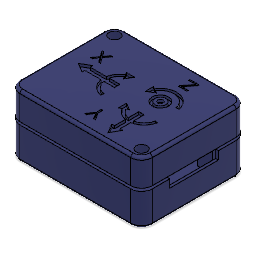
Sensor_Board_Box v9 (Autodesk Fusion 360 design; units mm, degrees)
Autodesk Fusion 360 part; units mm, degrees
sketch "Sketch1" plane through (0, 0, 0) normal (0, 1, 0) x (1, 0, 0)
  line L0 (17.5, -13.25) -> (-17.5, -13.25)
  line L1 (-17.5, -13.25) -> (-17.5, 13.25)
  line L2 (-17.5, 13.25) -> (17.5, 13.25)
  line L3 (17.5, 13.25) -> (17.5, -13.25)
  line L4 (17.5, -13.25) -> (-17.5, 13.25) construction
  line L5 (-17.5, -13.25) -> (17.5, 13.25) construction
  line L6 (-17.5, 13.25) -> (-20.689, 15.6646)
  circle A0 centre (-20.689, 15.6646) radius 1.35
  line L7 (-20.5, 19.5) -> (20.5, 19.5)
  line L8 (24.5, 15.5) -> (24.5, -15.5)
  line L9 (20.5, -19.5) -> (-20.5, -19.5)
  line L10 (-24.5, -15.5) -> (-24.5, 15.5)
  line L11 (-24.5, 19.5) -> (24.5, -19.5) construction
  line L12 (24.5, 19.5) -> (-24.5, -19.5) construction
  line L13 (-24.5, 15.5) -> (-24.5, 12.5)
  line L14 (-24.5, 12.5) -> (-21.5, 12.5)
  line L15 (-20.5, 19.5) -> (-17.5, 19.5)
  line L16 (-17.5, 19.5) -> (-17.5, 16.5)
  arc A1 (-21.5, 12.5) -> (-17.5, 16.5) centre (-21.5, 16.5) ccw
  arc A2 (-20.5, 19.5) -> (-24.5, 15.5) centre (-20.5, 15.5) ccw
  line L17 (24.5, -12.5) -> (21.5, -12.5)
  arc A3 (21.5, -12.5) -> (17.5, -16.5) centre (21.5, -16.5) ccw
  circle A4 centre (20.689, -15.6646) radius 1.35
  line L18 (17.5, -19.5) -> (17.5, -16.5)
  arc A5 (20.5, -19.5) -> (24.5, -15.5) centre (20.5, -15.5) ccw
  line L19 (23.5, -12.5) -> (23.5, 14.5)
  line L20 (23.5, 18.5) -> (-23.5, -18.5) construction
  line L21 (-23.5, 18.5) -> (23.5, -18.5) construction
  line L22 (19.5, 18.5) -> (-17.5, 18.5)
  line L23 (-23.5, 12.5) -> (-23.5, -14.5)
  line L24 (-19.5, -18.5) -> (17.5, -18.5)
  arc A6 (23.5, 14.5) -> (19.5, 18.5) centre (19.5, 14.5) ccw
  arc A7 (24.5, 15.5) -> (20.5, 19.5) centre (20.5, 15.5) ccw
  arc A8 (-23.5, -14.5) -> (-19.5, -18.5) centre (-19.5, -14.5) ccw
  arc A9 (-24.5, -15.5) -> (-20.5, -19.5) centre (-20.5, -15.5) ccw
  dimension "d1" = 35
  dimension "d2" = 26.5
  dimension "d3" = 4
  dimension "d4" = 2.7
  dimension "d5" = 49
  dimension "d6" = 39
  dimension "d7" = 7
  dimension "d8" = 3
  dimension "d9" = 7
  dimension "d10" = 3
  dimension "d11" = 4
  dimension "d13" = 180
  dimension "d14" = 47
  dimension "d15" = 37
  dimension "d16" = 4
  dimension "d17" = 4
  dimension "d18" = 4
  dimension "d19" = 4
  constraint perpendicular L0 L1
  constraint parallel L0 L2
  constraint parallel L1 L3
  constraint horizontal L0
  constraint coincident L4 origin
  constraint coincident L5 origin
  constraint parallel L4 L6
  constraint coincident L6.end A0.centre
  constraint perpendicular L7 L8
  constraint parallel L7 L9
  constraint parallel L8 L10
  constraint horizontal L7
  constraint coincident L11 origin
  constraint coincident L12 origin
  constraint perpendicular L7 L13
  constraint perpendicular L13 L14
  constraint perpendicular L13 L15
  constraint perpendicular L15 L16
  constraint tangent L16 A1
  constraint coincident L11.start L15
  constraint coincident L11.start L13
  constraint tangent L15 A2
  constraint tangent L13 A2
  constraint parallel L22 L24
  constraint horizontal L22
  constraint coincident L20 origin
  constraint coincident L21 origin
  constraint coincident L16 L22.end
  constraint coincident L14 L23.start
  constraint coincident L18 L24.end
  constraint coincident L17 L19.start
  constraint tangent L19 A6
  constraint tangent L22 A6
  constraint coincident L12.start L7
  constraint tangent L8 A7
  constraint tangent L7 A7
  constraint coincident L20.end L24
  constraint coincident L20.end L23
  constraint tangent L24 A8
  constraint tangent L23 A8
  constraint coincident L12.end L9
  constraint coincident L12.end L10
  constraint tangent L9 A9
  constraint tangent L10 A9
  measures "d1" distance of L1.end L2.end
  measures "d2" distance of L0.end L1.end
  measures "d3" distance of L1.end L6.end
  measures "d4" diameter of A0
  measures "d5" distance of L11.end L12.end
  measures "d6" distance of L12.start L11.end
  measures "d7" distance of L11.start L13.end
  measures "d8" distance of L13.end L14.end
  measures "d9" distance of L11.start L15.end
  measures "d10" distance of L15.end L16.end
  measures "d11" radius of A2
  measures "d14" distance of L20.end L21.end
  measures "d15" distance of L21.start L20.end
  measures "d16" radius of A6
  measures "d17" radius of A7
  measures "d18" radius of A8
  measures "d19" radius of A9
sketch "Sketch1 (2)" plane through (0, 0, 0) normal (0, 1, 0) x (1, 0, 0) in component "Bottom"
  line L0 (-24.5, 19.5) -> (24.5, -19.5) construction
  line L1 (-23.5, 18.5) -> (23.5, -18.5) construction
  circle A0 centre (-20.689, 15.6646) radius 1.35
  line L2 (-17.5, 13.25) -> (-20.689, 15.6646) construction
  arc A1 (-21.5, 12.5) -> (-17.5, 16.5) centre (-21.5, 16.5) ccw
  line L3 (-17.5, 13.25) -> (17.5, 13.25)
  line L4 (17.5, -13.25) -> (-17.5, 13.25) construction
  line L5 (-17.5, -13.25) -> (-17.5, 13.25)
  line L6 (19.5, 18.5) -> (-17.5, 18.5)
  line L7 (-20.5, 19.5) -> (20.5, 19.5)
  line L8 (24.5, 19.5) -> (-24.5, -19.5) construction
  line L9 (23.5, 18.5) -> (-23.5, -18.5) construction
  line L10 (23.5, -12.5) -> (23.5, 14.5)
  line L11 (24.5, 15.5) -> (24.5, -15.5)
  line L12 (17.5, 13.25) -> (17.5, -13.25)
  arc A2 (21.5, -12.5) -> (17.5, -16.5) centre (21.5, -16.5) ccw
  line L13 (17.5, -13.25) -> (-17.5, -13.25)
  circle A3 centre (20.689, -15.6646) radius 1.35
  arc A4 (20.5, -19.5) -> (24.5, -15.5) centre (20.5, -15.5) ccw
  line L14 (24.5, -12.5) -> (21.5, -12.5)
  line L15 (20.5, -19.5) -> (-20.5, -19.5)
  line L16 (-19.5, -18.5) -> (17.5, -18.5)
  line L17 (17.5, -19.5) -> (17.5, -16.5)
  line L18 (-17.5, -13.25) -> (17.5, 13.25) construction
  line L19 (-23.5, 12.5) -> (-23.5, -14.5)
  line L20 (-24.5, -15.5) -> (-24.5, 15.5)
  line L21 (-24.5, 12.5) -> (-21.5, 12.5)
  arc A5 (-20.5, 19.5) -> (-24.5, 15.5) centre (-20.5, 15.5) ccw
  line L22 (-17.5, 19.5) -> (-17.5, 16.5)
  arc A6 (-24.5, -15.5) -> (-20.5, -19.5) centre (-20.5, -15.5) ccw
  arc A7 (-23.5, -14.5) -> (-19.5, -18.5) centre (-19.5, -14.5) ccw
  arc A8 (23.5, 14.5) -> (19.5, 18.5) centre (19.5, 14.5) ccw
  arc A9 (24.5, 15.5) -> (20.5, 19.5) centre (20.5, 15.5) ccw
  point P0 (-23.5, 18.5)
  point P1 (-24.5, 19.5)
  point P2 (-21.5, 16.5)
  point P3 (-20.689, 15.6646)
  point P4 (-20.689, 15.6646)
  point P5 (-20.5, 15.5)
  point P6 (-17.5, 13.25)
  point P7 (17.5, -13.25)
  point P8 (20.5, -15.5)
  point P9 (20.689, -15.6646)
  point P10 (24.5, -19.5)
  point P11 (23.5, -18.5)
  point P12 (24.5, -15.5)
  point P13 (24.5, -12.5)
  point P14 (23.5, -12.5)
  point P15 (21.5, -12.5)
  point P16 (21.5, -16.5)
  point P17 (20.5, -19.5)
  point P18 (17.5, -18.5)
  point P19 (17.5, -19.5)
  point P20 (-24.5, -19.5)
  point P21 (-21.5, 12.5)
  point P22 (-23.5, 12.5)
  point P23 (-24.5, 15.5)
  point P24 (-17.5, 19.5)
  point P25 (-20.5, 19.5)
  point P26 (-17.5, 18.5)
  point P27 (-17.5, 16.5)
  point P28 (17.5, 13.25)
  point P29 (-17.5, -13.25)
  point P30 (-23.5, -18.5)
  point P31 (17.5, -16.5)
extrude "Extrude1" add sketch "Sketch1 (2)" along normal blind 2 contours A0 | A1 L7 L20 L21 A5 L22 | A1 L6 L10 A2 L14 L16 L17 L19 L21 L22 A7 A8 | L15 L16 L17 L19 L20 L21 A6 A7 | L6 L7 L10 L11 L14 L22 A8 A9 | L11 A2 A4 L14 L15 L17 | L3 L5 L12 L13 | A3 makes body 1 in component "Bottom"
extrude "Extrude2" add sketch "Sketch1 (2)" along normal blind 3 contours A1 L6 L10 A2 L14 L16 L17 L19 L21 L22 A7 A8 bodies 1 in component "Bottom"
extrude "Extrude3" add 1 faces at (23.1667, 2, 13.5) along direction (0, 1, 0) blind 10 on bodies 1 bodies 1 in component "Bottom"
extrude "Extrude4" cut sketch "Sketch1 (2)" along normal blind 29 from surface at 3 contours A0 | A3 bodies 1 in component "Bottom"
sketch "Sketch1 (3)" plane through (0, 0, 0) normal (0, 0, 1) x (1, 0, 0) in component "Top"
  line L0 (17.5, 3) -> (17.5, 2)
  line L1 (17.5, 2) -> (-17.5, 2)
  line L2 (-17.5, 2) -> (-17.5, 3)
  line L3 (-17.5, 3) -> (-23.5, 3)
  line L4 (-23.5, 3) -> (-23.5, 12)
  line L5 (-23.5, 12) -> (-24.5, 12)
  line L6 (-24.5, 12) -> (-24.5, 0)
  line L7 (-24.5, 0) -> (24.5, 0)
  line L8 (24.5, 0) -> (24.5, 12)
  line L9 (24.5, 12) -> (23.5, 12)
  line L10 (23.5, 12) -> (23.5, 3)
  line L11 (23.5, 3) -> (17.5, 3)
  line L12 (0, 2) -> (0, 22) construction
  dimension "d30" = 20
  constraint vertical L12
  constraint midpoint L1 L12.start
  measures "d30" distance of L12.start L12.end
sketch "Sketch2" plane through (0, 12, 0) normal (0, 1, 0) x (-1, 0, 0) in component "Top"
  line L0 (-17.5, -13.25) -> (-17.5, 13.25) construction
  line L1 (-17.5, 13.25) -> (17.5, 13.25) construction
  line L2 (17.5, -13.25) -> (-17.5, -13.25) construction
  line L3 (-23.5, 12.5) -> (-23.5, -14.5) construction
  arc A0 (-23.5, -14.5) -> (-19.5, -18.5) centre (-19.5, -14.5) ccw construction
  line L4 (-19.5, -18.5) -> (17.5, -18.5) construction
  line L5 (17.5, -18.5) -> (17.5, -16.5) construction
  arc A1 (21.5, -12.5) -> (17.5, -16.5) centre (21.5, -16.5) ccw construction
  line L6 (21.5, -12.5) -> (23.5, -12.5) construction
  line L7 (23.5, -12.5) -> (23.5, 14.5) construction
  arc A2 (23.5, 14.5) -> (19.5, 18.5) centre (19.5, 14.5) ccw construction
  line L8 (19.5, 18.5) -> (-17.5, 18.5) construction
  line L9 (-17.5, 18.5) -> (-17.5, 16.5) construction
  arc A3 (-21.5, 12.5) -> (-17.5, 16.5) centre (-21.5, 16.5) ccw construction
  line L10 (-21.5, 12.5) -> (-23.5, 12.5) construction
  circle A4 centre (20.689, -15.6646) radius 1.35 construction
  circle A5 centre (-20.689, 15.6646) radius 1.35 construction
  arc A6 (21.5, -12.5) -> (17.5, -16.5) centre (21.5, -16.5) ccw construction
  line L11 (17.5, -16.5) -> (17.5, -18.5) construction
  line L12 (17.5, -18.5) -> (-19.5, -18.5) construction
  arc A7 (-19.5, -18.5) -> (-23.5, -14.5) centre (-19.5, -14.5) cw construction
  line L13 (-23.5, -14.5) -> (-23.5, 12.5) construction
  line L14 (-23.5, 12.5) -> (-21.5, 12.5) construction
  arc A8 (-21.5, 12.5) -> (-17.5, 16.5) centre (-21.5, 16.5) ccw construction
  line L15 (-17.5, 16.5) -> (-17.5, 18.5) construction
  line L16 (-17.5, 18.5) -> (19.5, 18.5) construction
  arc A9 (19.5, 18.5) -> (23.5, 14.5) centre (19.5, 14.5) cw construction
  line L17 (23.5, 14.5) -> (23.5, -12.5) construction
  line L18 (23.5, -12.5) -> (21.5, -12.5) construction
  line L19 (17.5, 13.25) -> (17.5, -13.25) construction
  line L20 (17.5, -13.25) -> (-17.5, -13.25) construction
  line L21 (-17.5, -13.25) -> (-17.5, 13.25) construction
  line L22 (-17.5, 13.25) -> (17.5, 13.25) construction
  line L23 (20.5, 19.5) -> (-20.5, 19.5)
  arc A10 (-20.5, 19.5) -> (-24.5, 15.5) centre (-20.5, 15.5) ccw
  line L24 (-24.5, 15.5) -> (-24.5, -15.5)
  arc A11 (-24.5, -15.5) -> (-20.5, -19.5) centre (-20.5, -15.5) ccw
  line L25 (-20.5, -19.5) -> (20.5, -19.5)
  arc A12 (20.5, -19.5) -> (24.5, -15.5) centre (20.5, -15.5) ccw
  line L26 (24.5, -15.5) -> (24.5, 15.5)
  arc A13 (24.5, 15.5) -> (20.5, 19.5) centre (20.5, 15.5) ccw
  circle A14 centre (20.689, -15.6646) radius 2
  line L27 (17.5, -18.5) -> (17, -18.5) construction
  line L28 (17, -18.5) -> (17, -18)
  line L29 (23.5, -12.5) -> (23.5, -12) construction
  line L30 (23.5, -12) -> (23, -12)
  line L31 (17.5, -13.25) -> (17.5, -10.75) construction
  line L32 (17.5, -13.25) -> (15, -13.25) construction
  arc A15 (21, -12) -> (17, -16) centre (21, -16) ccw
  line L33 (15, -13.25) -> (17.5, -10.75)
  line L34 (23.5, -12.5) -> (23, -12.5) construction
  line L35 (23, -12.5) -> (23, -12) construction
  line L36 (23, -12) -> (23.5, -12) construction
  line L37 (23.5, -12) -> (23.5, -12.5) construction
  line L38 (23.5, 14.5) -> (23, 14.5) construction
  line L39 (23, 14.5) -> (23, 14) construction
  line L40 (23, 14) -> (23.5, 14) construction
  line L41 (23.5, 14) -> (23.5, 14.5) construction
  line L42 (19.5, 18.5) -> (19, 18.5) construction
  line L43 (19, 18.5) -> (19, 18) construction
  line L44 (19, 18) -> (19.5, 18)
  line L45 (19.5, 18) -> (19.5, 18.5) construction
  arc A16 (23, 14.5) -> (19.5, 18) centre (19.5, 14.5) ccw
  line L46 (21, -12) -> (23, -12)
  line L47 (23, -12) -> (23, 14.5)
  line L48 (17.5, -18.5) -> (17, -18.5) construction
  line L49 (17, -18.5) -> (17, -18) construction
  line L50 (17, -18) -> (17.5, -18) construction
  line L51 (17.5, -18) -> (17.5, -18.5) construction
  line L52 (17, -16) -> (17, -18)
  line L53 (17.5, -10.75) -> (23, -10.75)
  line L54 (15, -13.25) -> (15, -18)
  line L55 (15, -18) -> (17, -18)
  line L56 (-17.5, 0) -> (17.5, 0)
  line L57 (15, 13.25) -> (17.5, 10.75)
  line L58 (17.5, 13.25) -> (15, 13.25) construction
  line L59 (17.5, 13.25) -> (17.5, 10.75) construction
  line L60 (17.5, 10.75) -> (23, 10.75)
  line L61 (15, 13.25) -> (15, 18)
  line L62 (15, 18) -> (19, 18)
  line L63 (23, 0) -> (21, 0) construction
  line L64 (21, 0) -> (21, -10.75)
  line L65 (21, 0) -> (21, 10.75)
  circle A17 centre (-20.689, 15.6646) radius 2
  line L66 (-17, 16) -> (-17, 18)
  arc A18 (-21, 12) -> (-17, 16) centre (-21, 16) ccw
  line L67 (-21, 12) -> (-23, 12)
  line L68 (-23, 12) -> (-23, -14.5)
  arc A19 (-23, -14.5) -> (-19.5, -18) centre (-19.5, -14.5) ccw
  line L69 (-17, 18) -> (15, 18)
  line L70 (-19.5, -18) -> (15, -18)
  line L71 (-17.5, -13.25) -> (-17.5, -8.25) construction
  line L72 (-17.5, -13.25) -> (-12.5, -13.25) construction
  line L73 (-17.5, -8.25) -> (-12.5, -13.25)
  line L74 (-12.5, -13.25) -> (-12.5, -18)
  line L75 (-17.5, -8.25) -> (-23, -8.25)
  line L76 (-17.5, 8.25) -> (-12.5, 13.25)
  line L77 (-17.5, 13.25) -> (-12.5, 13.25) construction
  line L78 (-17.5, 13.25) -> (-17.5, 8.25) construction
  line L79 (-17.5, 8.25) -> (-23, 8.25)
  line L80 (-12.5, 13.25) -> (-12.5, 18)
  line L81 (-23, 0) -> (-21, 0) construction
  line L82 (-12.5, -18) -> (-12.5, -16) construction
  line L83 (-12.5, -16) -> (15, -16)
  line L84 (15, 18) -> (15, 16) construction
  line L85 (15, 16) -> (-12.5, 16)
  line L86 (-21, 0) -> (-21, -8.25)
  line L87 (-21, 0) -> (-21, 8.25)
  circle A20 centre (20.689, -15.6646) radius 1.35
  circle A21 centre (-20.689, 15.6646) radius 1.35
  arc A22 (-20.5, 19.5) -> (-24.5, 15.5) centre (-20.5, 15.5) ccw
  line L88 (-24.5, 15.5) -> (-24.5, -15.5)
  arc A23 (-24.5, -15.5) -> (-20.5, -19.5) centre (-20.5, -15.5) ccw
  line L89 (-20.5, -19.5) -> (20.5, -19.5)
  arc A24 (20.5, -19.5) -> (24.5, -15.5) centre (20.5, -15.5) ccw
  line L90 (24.5, -15.5) -> (24.5, 15.5)
  arc A25 (24.5, 15.5) -> (20.5, 19.5) centre (20.5, 15.5) ccw
  line L91 (20.5, 19.5) -> (-20.5, 19.5)
  line L92 (-23.5, 12.5) -> (-21.5, 12.5) construction
  arc A26 (-21.5, 12.5) -> (-17.5, 16.5) centre (-21.5, 16.5) ccw construction
  line L93 (-17.5, 16.5) -> (-17.5, 18.5) construction
  line L94 (-17.5, 18.5) -> (19.5, 18.5) construction
  arc A27 (23.5, 14.5) -> (19.5, 18.5) centre (19.5, 14.5) ccw construction
  line L95 (23.5, 14.5) -> (23.5, -12.5) construction
  line L96 (23.5, -12.5) -> (21.5, -12.5) construction
  arc A28 (21.5, -12.5) -> (17.5, -16.5) centre (21.5, -16.5) ccw construction
  line L97 (17.5, -16.5) -> (17.5, -18.5) construction
  line L98 (17.5, -18.5) -> (-19.5, -18.5) construction
  arc A29 (-23.5, -14.5) -> (-19.5, -18.5) centre (-19.5, -14.5) ccw construction
  line L99 (-23.5, -14.5) -> (-23.5, 12.5) construction
  line L100 (17.5, 0) -> (0.5, 0) construction
  line L101 (17.5, 0) -> (24.5, 0)
  dimension "d31" = 4
  dimension "d32" = 0.5
  dimension "d33" = 2.5
  dimension "d34" = 0.5
  dimension "d35" = 2.5
  dimension "d36" = 2.5
  dimension "d37" = 2.5
  dimension "d38" = 0.5
  dimension "d39" = 0.5
  dimension "d40" = 0.5
  dimension "d41" = 0.5
  dimension "d42" = 0.5
  dimension "d43" = 0.5
  dimension "d44" = 0.5
  dimension "d45" = 0.5
  dimension "d46" = 2
  dimension "d50" = 5
  dimension "d51" = 5
  dimension "d52" = 2
  dimension "d53" = 2
  dimension "d54" = 2
  dimension "d81" = 17
  constraint concentric A4 A14
  constraint coincident L4.end L5.start
  constraint perpendicular L11 L27
  constraint perpendicular L4 L28
  constraint coincident L6.end L7.start
  constraint perpendicular L18 L29
  constraint perpendicular L7 L30
  constraint coincident L2.start L19.end
  constraint perpendicular L2 L31
  constraint perpendicular L19 L32
  constraint tangent L30 A15
  constraint horizontal L34
  constraint vertical L35
  constraint horizontal L36
  constraint vertical L37
  constraint horizontal L38
  constraint vertical L39
  constraint horizontal L40
  constraint vertical L41
  constraint coincident L7.end A2.start
  constraint horizontal L42
  constraint vertical L43
  constraint horizontal L44
  constraint vertical L45
  constraint coincident A2.end L8.start
  constraint tangent L39 A16
  constraint tangent A15 L46
  constraint horizontal L48
  constraint vertical L49
  constraint horizontal L50
  constraint vertical L51
  constraint tangent A15 L52
  constraint coincident L47 L53.end
  constraint perpendicular L47 L53
  constraint perpendicular L32 L54
  constraint perpendicular L49 L55
  constraint symmetric L2.start L56 L1.end
  constraint symmetric L31.end L56 L57.end
  constraint symmetric L32.end L56 L57.start
  constraint coincident L47 L60.end
  constraint perpendicular L47 L60
  constraint perpendicular L44 L61
  constraint perpendicular L43 L62
  constraint coincident L47 L63.start
  constraint perpendicular L47 L63
  constraint coincident L53 L64.end
  constraint perpendicular L53 L64
  constraint coincident L60 L65.end
  constraint perpendicular L60 L65
  constraint perpendicular L61 L69
  constraint tangent A19 L70
  constraint coincident L0.start L2.end
  constraint perpendicular L20 L71
  constraint perpendicular L21 L72
  constraint coincident L70 L74.end
  constraint perpendicular L70 L74
  constraint coincident L68 L75.end
  constraint perpendicular L68 L75
  constraint symmetric L56 L0.start L0.end
  constraint symmetric L56 L71.end L76.start
  constraint symmetric L56 L72.end L76.end
  constraint coincident L68 L79.end
  constraint perpendicular L68 L79
  constraint coincident L69 L80.end
  constraint perpendicular L69 L80
  constraint coincident L68 L81.start
  constraint perpendicular L68 L81
  constraint perpendicular L70 L82
  constraint coincident L54 L83.end
  constraint perpendicular L54 L83
  constraint perpendicular L62 L84
  constraint coincident L80 L85.end
  constraint perpendicular L80 L85
  constraint coincident L75 L86.end
  constraint perpendicular L75 L86
  constraint coincident L79 L87.end
  constraint perpendicular L79 L87
  constraint perpendicular L19 L100
  constraint midpoint L90 L101.end
  measures "d31" diameter of A14
  measures "d32" distance of L4.end L27.end
  measures "d33" distance of L27.end A15.end
  measures "d34" distance of L6.end L29.end
  measures "d35" distance of L29.end A15.start
  measures "d36" distance of L2.start L31.end
  measures "d37" distance of L2.start L32.end
  measures "d38" distance of L6.end L34.end
  measures "d39" distance of L6.end L29.end
  measures "d40" distance of L7.end L38.end
  measures "d41" distance of L7.end L40.end
  measures "d42" distance of A2.end L42.end
  measures "d43" distance of A2.end L44.end
  measures "d44" distance of L4.end L27.end
  measures "d45" distance of L4.end L50.end
  measures "d46" distance of L63.start L63.end
  measures "d50" distance of L0.start L71.end
  measures "d51" distance of L0.start L72.end
  measures "d52" distance of L81.start L81.end
  measures "d53" distance of L74.end L82.end
  measures "d54" distance of L61.end L84.end
  measures "d81" distance of L56.end L100.end
sketch "Sketch3" plane through (-24.5, 0, 0) normal (-1, 0, 0) x (0, 0, 1) in component "Bottom"
  line L0 (-15.5, 0) -> (15.5, 0)
  line L1 (15.5, 0) -> (15.5, 12)
  line L2 (15.5, 12) -> (-15.5, 12) construction
  line L3 (-15.5, 12) -> (-15.5, 0)
  line L4 (14.5, 3) -> (-12.5, 3)
  line L5 (-12.5, 3) -> (-12.5, 12)
  line L6 (-12.5, 12) -> (14.5, 12) construction
  line L7 (14.5, 12) -> (14.5, 3)
  line L8 (13.25, 2) -> (-13.25, 2)
  line L9 (-13.25, 2) -> (-13.25, 3)
  line L10 (-13.25, 3) -> (13.25, 3)
  line L11 (13.25, 3) -> (13.25, 2)
  line L12 (0, 2) -> (0, 9) construction
  line L13 (0, 9) -> (9, 9) construction
  line L14 (9, 9) -> (-9, 9)
  line L15 (-9, 9) -> (-9, 13)
  line L16 (-9, 13) -> (9, 13)
  line L17 (9, 13) -> (9, 9)
  dimension "d55" = 7
  dimension "d56" = 9
  dimension "d57" = 18
  dimension "d58" = 4
  constraint midpoint L8 L12.start
  constraint perpendicular L8 L12
  constraint horizontal L13
  constraint horizontal L14
  constraint vertical L15
  constraint horizontal L16
  constraint vertical L17
  measures "d55" distance of L12.start L12.end
  measures "d56" distance of L12.end L13.end
  measures "d57" distance of L13.end L14.end
  measures "d58" distance of L13.end L16.end
extrude "Extrude1'" add sketch "Sketch2" along normal blind 9 from surface at 1 separate body contours L23 A10 L24 A11 L25 A12 L26 A13 A22 L88 A23 L89 A24 L90 A25 L91 | A15 L33 L46 L47 L52 L53 L54 L55 | L47 L53 L64 L101 | L54 L70 L74 L83 | L47 L60 L65 L101 | L68 A19 L70 L73 L74 L75 | L44 A16 L47 L57 L60 L61 L62 | L68 L75 L79 L86 L87 | L66 A18 L67 L68 L69 L76 L79 L80 | L61 L69 L80 L85 makes body 2 in component "Top"
extrude "Extrude2'" add sketch "Sketch2" along normal blind 1 contours A15 L33 L46 L47 L52 L53 L54 L55 | L47 L53 L64 L101 | L54 L70 L74 L83 | L47 L60 L65 L101 | L68 A19 L70 L73 L74 L75 | L44 A16 L47 L57 L60 L61 L62 | L68 L75 L79 L86 L87 | L66 A18 L67 L68 L69 L76 L79 L80 | L61 L69 L80 L85 bodies 2 in component "Top"
extrude "Extrude3'" add sketch "Sketch2" along normal blind -8 and the other way blind -4 contours A15 L33 L46 L47 L52 L53 L54 L55 | L68 A19 L70 L73 L74 L75 | L44 A16 L47 L57 L60 L61 L62 | L66 A18 L67 L68 L69 L76 L79 L80 bodies 2 in component "Top"
extrude "Extrude4'" add sketch "Sketch2" along normal blind 3 and the other way blind 3 contours L47 L53 L64 L101 | L54 L70 L74 L83 | L47 L60 L65 L101 | L68 L75 L79 L86 L87 | L61 L69 L80 L85 bodies 2 in component "Top"
extrude "Extrude5" add 1 faces at (16.8333, 22, -13.6667) along direction (0, 1, 0) blind 1 on bodies 2 bodies 2 in component "Top"
extrude "Extrude6" add sketch "Sketch2" along normal blind 2 from surface at 9 contours L33 L53 L54 L57 L60 L61 L64 L65 L73 L74 L75 L76 L79 L80 L83 L85 L86 L87 bodies 2 in component "Top"
fillet "Fillet1" radius 1 8 edges at (23.3284, 23, -18.3284) (0, 23, -19.5) (-23.3284, 23, -18.3284) (-24.5, 23, 0) (-23.3284, 23, 18.3284) (0, 23, 19.5) (23.3284, 23, 18.3284) (24.5, 23, 0) on bodies 2 in component "Top"
fillet "Fillet1'" radius 1 8 edges at (23.3284, 0, 18.3284) (0, 0, 19.5) (-23.3284, 0, 18.3284) (-24.5, 0, 0) (-23.3284, 0, -18.3284) (0, 0, -19.5) (23.3284, 0, -18.3284) (24.5, 0, 0) on bodies 1 in component "Bottom"
extrude "Extrude6'" cut sketch "Sketch3" against normal blind 51 contours L14 L15 L16 L17 bodies 1 in component "Bottom"
sketch "Sketch5" plane through (23, 0, 0) normal (1, 0, 0) x (0, 0, -1) in component "Top"
  line L0 (14.5, 13) -> (-12, 13)
  line L1 (-12, 13) -> (-12, 4)
  line L2 (-12, 4) -> (-8.25, 4)
  line L3 (-8.25, 4) -> (-8.25, 9)
  line L4 (-8.25, 9) -> (8.25, 9)
  line L5 (8.25, 9) -> (8.25, 4)
  line L6 (8.25, 4) -> (14.5, 4)
  line L7 (14.5, 4) -> (14.5, 13)
  line L8 (-8.25, 9) -> (-8.25, 13)
  line L9 (8.25, 9) -> (8.25, 13)
  constraint coincident L3.end L4.start
  constraint coincident L0 L8.end
  constraint perpendicular L0 L8
  constraint coincident L4.end L5.start
  constraint coincident L0 L9.end
  constraint perpendicular L0 L9
extrude "Extrude8" cut sketch "Sketch5" against normal blind 53 contours L0 L4 L8 L9 bodies 2 in component "Top"
sketch "Sketch6" plane through (0, 23, 0) normal (0, 1, 0) x (-1, 0, 0) in component "Top"
  circle A0 centre (20.689, -15.6646) radius 2
  circle A1 centre (-20.689, 15.6646) radius 2
  arc A2 (-23.5, -15.5) -> (-20.5, -18.5) centre (-20.5, -15.5) ccw
  line L0 (-20.5, -18.5) -> (20.5, -18.5)
  arc A3 (20.5, -18.5) -> (23.5, -15.5) centre (20.5, -15.5) ccw
  line L1 (23.5, -15.5) -> (23.5, 15.5)
  arc A4 (23.5, 15.5) -> (20.5, 18.5) centre (20.5, 15.5) ccw
  line L2 (20.5, 18.5) -> (-20.5, 18.5)
  arc A5 (-20.5, 18.5) -> (-23.5, 15.5) centre (-20.5, 15.5) ccw
  line L3 (-23.5, 15.5) -> (-23.5, -15.5)
  line L4 (-9, -3) -> (-14.9088, -4.0419) construction
  line L5 (-9, -3) -> (-9, -8) construction
  line L6 (-9, -3) -> (-4.6699, -5.5) construction
  line L7 (-9, -3) -> (-9, -8) construction
  line L8 (-9, -3) -> (-9, -9) construction
  line L9 (-2.9378, -6.5) -> (-2.9378, -3.5)
  line L10 (-9, -3) -> (-13.924, -3.8682) construction
  line L11 (-5.5359, -5) -> (-2.9378, -3.5)
  line L12 (-9, -6) -> (-9, -8)
  arc A6 (-9, -8) -> (-4.6699, -5.5) centre (-9, -3) ccw
  line L13 (-9, -3) -> (-9, -6) construction
  line L14 (-9, -8) -> (-9, -9) construction
  line L15 (-13.924, -3.8682) -> (-14.9088, -4.0419)
  line L16 (-3.8038, -6) -> (-2.9378, -6.5)
  circle A7 centre (-9, -3) radius 1
  arc A8 (-14.9088, -4.0419) -> (-9, -9) centre (-9, -3) ccw
  line L17 (-4.6699, -5.5) -> (-5.5359, -5)
  circle A9 centre (-9, -3) radius 3
  arc A10 (-9, -9) -> (-3.8038, -6) centre (-9, -3) ccw
  arc A11 (-13.924, -3.8682) -> (-9, -8) centre (-9, -3) ccw
  line L18 (-9, -3) -> (-9, -9) construction
  line L19 (-9, -3) -> (-3.8038, -6) construction
  circle A12 centre (-9, -3) radius 2
  line L20 (-10.8275, -15.5029) -> (-7.432, -15.5029) construction
  line L21 (-7.432, -15.5029) -> (-7.432, -9.5029) construction
  line L22 (-7.432, -9.5029) -> (-10.8275, -9.5029) construction
  line L23 (-10.8275, -9.5029) -> (-10.8275, -15.5029) construction
  line L24 (0, 0) -> (4, 0) construction
  line L25 (4, 0) -> (4, 1)
  line L26 (4, 0) -> (4, -1)
  line L27 (4, 1) -> (15, 1)
  line L28 (15, 1) -> (15, 2)
  line L29 (4, -1) -> (15, -1)
  line L30 (15, -1) -> (15, -2)
  line L31 (15, 2) -> (18.4641, 0)
  line L32 (15, -2) -> (18.4641, 0)
  line L33 (14.1725, -8.5029) -> (18.11, -8.5029) construction
  line L34 (18.11, -8.5029) -> (18.11, -2.5029) construction
  line L35 (18.11, -2.5029) -> (14.1725, -2.5029) construction
  line L36 (14.1725, -2.5029) -> (14.1725, -8.5029) construction
  arc A13 (5.5622, -4.2679) -> (7.6024, -2.0322) centre (3.0622, 0.0622) ccw
  line L37 (6.5622, -6) -> (3.5622, -6)
  line L38 (3.9304, 4.9862) -> (4.1041, 5.971)
  arc A14 (6.0622, -5.134) -> (8.5104, -2.4511) centre (3.0622, 0.0622) ccw
  line L39 (6.0622, -5.134) -> (6.5622, -6)
  line L40 (5.0622, -3.4019) -> (3.5622, -6)
  line L41 (5.5622, -4.2679) -> (5.0622, -3.4019)
  line L42 (-10.2679, 4.2679) -> (-10.2679, 13.2679)
  line L43 (-11.2679, 13.2679) -> (-9.2679, 16.7321)
  line L44 (-10.2679, 13.2679) -> (-11.2679, 13.2679)
  line L45 (-8.2679, 4.2679) -> (-8.2679, 13.2679)
  line L46 (-8.2679, 13.2679) -> (-7.2679, 13.2679)
  arc A15 (-4.134, 6.3301) -> (-6.8169, 8.7784) centre (-9.3301, 3.3301) ccw
  line L47 (-14.2542, 4.1984) -> (-15.239, 4.372)
  line L48 (-9.2679, 4.2679) -> (-8.2679, 4.2679)
  line L49 (-5.866, 5.3301) -> (-3.2679, 3.8301)
  arc A16 (-5, 5.8301) -> (-7.2358, 7.8704) centre (-9.3301, 3.3301) ccw
  line L50 (-7.2679, 13.2679) -> (-9.2679, 16.7321)
  line L51 (-9.2679, 4.2679) -> (-10.2679, 4.2679)
  line L52 (-5, 5.8301) -> (-5.866, 5.3301)
  line L53 (-3.2679, 6.8301) -> (-3.2679, 3.8301)
  line L54 (-4.134, 6.3301) -> (-3.2679, 6.8301)
  line L55 (-2.8275, 10.4971) -> (1.11, 10.4971) construction
  line L56 (1.11, 10.4971) -> (1.11, 16.4971) construction
  line L57 (1.11, 16.4971) -> (-2.8275, 16.4971) construction
  line L58 (-2.8275, 16.4971) -> (-2.8275, 10.4971) construction
  arc A17 (7.6024, -2.0322) -> (7.9481, -1) centre (3.0622, 0.0622) ccw
  arc A18 (7.9734, 1) -> (3.9304, 4.9862) centre (3.0622, 0.0622) ccw
  arc A19 (7.9481, -1) -> (7.9734, 1) centre (3.0622, 0.0622) ccw construction
  arc A20 (8.5104, -2.4511) -> (8.9674, -1) centre (3.0622, 0.0622) ccw
  arc A21 (8.9884, 1) -> (4.1041, 5.971) centre (3.0622, 0.0622) ccw
  arc A22 (8.9674, -1) -> (8.9884, 1) centre (3.0622, 0.0622) ccw construction
  arc A23 (-6.8169, 8.7784) -> (-8.2679, 9.2354) centre (-9.3301, 3.3301) ccw
  arc A24 (-10.2679, 9.2564) -> (-15.239, 4.372) centre (-9.3301, 3.3301) ccw
  arc A25 (-8.2679, 9.2354) -> (-10.2679, 9.2564) centre (-9.3301, 3.3301) ccw construction
  arc A26 (-7.2358, 7.8704) -> (-8.2679, 8.216) centre (-9.3301, 3.3301) ccw
  arc A27 (-10.2679, 8.2414) -> (-14.2542, 4.1984) centre (-9.3301, 3.3301) ccw
  arc A28 (-8.2679, 8.216) -> (-10.2679, 8.2414) centre (-9.3301, 3.3301) ccw construction
  dimension "d101" = 2
  dimension "d102" = 4
  dimension "d103" = 6
  dimension "d104" = 2
  dimension "d105" = 80
  dimension "d106" = 60
  dimension "d107" = 1
  dimension "d108" = 80
  dimension "d109" = 60
  dimension "d110" = 1
  dimension "d111" = 1
  dimension "d112" = 4
  dimension "d113" = 1
  dimension "d114" = 1
  dimension "d115" = 11
  dimension "d116" = 1
  dimension "d117" = 11
  dimension "d118" = 1
  dimension "d122" = 1
  dimension "d123" = 1
  dimension "d125" = 1
  dimension "d127" = 1
  text T0 "Z" font "Arial" height 6 align ink ink in box 0 x 0 at (-10.8275, -15.5029) x (1, 0) y (0, 1) spacing 1 height is em
  text T1 "X" font "Arial" height 6 align ink ink in box 0 x 0 at (14.1725, -8.5029) x (1, 0) y (0, 1) spacing 1 height is em
  text T2 "Y" font "Arial" height 6 align ink ink in box 0 x 0 at (-2.8275, 10.4971) x (1, 0) y (0, 1) spacing 1 height is em
  constraint concentric A7 A12
  constraint concentric A7 A9
  constraint coincident L4.start L5.start
  constraint coincident L12.start A9
  constraint vertical L13
  constraint parallel L12 L13
  constraint parallel L5 L14
  constraint parallel L6 L17
  constraint parallel L16 L19
  constraint perpendicular L20 L21
  constraint parallel L20 L22
  constraint parallel L21 L23
  constraint coincident L24.start origin
  constraint horizontal L24
  constraint perpendicular L24 L25
  constraint perpendicular L24 L26
  constraint perpendicular L25 L27
  constraint perpendicular L27 L28
  constraint perpendicular L26 L29
  constraint perpendicular L29 L30
  constraint perpendicular L33 L34
  constraint parallel L33 L35
  constraint parallel L34 L36
  constraint perpendicular L42 L51
  constraint perpendicular L42 L44
  constraint perpendicular L45 L48
  constraint perpendicular L55 L56
  constraint parallel L55 L57
  constraint parallel L56 L58
  constraint coincident L29 A17.end
  constraint coincident L27 A18.start
  constraint concentric A17 A18
  constraint concentric A17 A19
  constraint coincident L29 A20.end
  constraint coincident L27 A21.start
  constraint concentric A20 A21
  constraint concentric A20 A22
  constraint coincident L45 A23.end
  constraint coincident L42 A24.start
  constraint concentric A23 A24
  constraint concentric A23 A25
  constraint coincident L45 A26.end
  constraint coincident L42 A27.start
  constraint concentric A26 A27
  constraint concentric A26 A28
  measures "d101" diameter of A7
  measures "d102" diameter of A12
  measures "d103" diameter of A9
  measures "d104" distance of L12.start L5.end
  measures "d105" angle of L5 L10
  measures "d106" angle of L6 L7
  measures "d107" distance of L8.end L5.end
  measures "d108" angle of L4 L8
  measures "d109" angle of L18 L19
  measures "d110" distance of L6.end L11.start
  measures "d111" distance of L16.start L9.start
  measures "d112" distance of L24.start L24.end
  measures "d113" distance of L24.end L25.end
  measures "d114" distance of L24.end L26.end
  measures "d115" distance of L25.end L27.end
  measures "d116" distance of L27.end L28.end
  measures "d117" distance of L26.end L29.end
  measures "d118" distance of L29.end L30.end
  measures "d122" distance of L48.start L42.start
  measures "d123" distance of L45.start L48.start
  measures "d125" distance of L43.start L42.end
  measures "d127" distance of L46.end L45.end
extrude "Extrude9" cut sketch "Sketch6" sketch "Sketch6" against normal blind 1 contours L9 L11 A6 L15 L16 A8 L17 A10 A11 | A7 | A9 | L25 L26 L27 L28 L29 L30 L31 L32 | L27 L38 A18 A21 | L29 A13 L37 A14 L39 L40 L41 A17 A20 | L42 L43 L44 L45 L46 L48 L50 L51 | L42 L47 A24 A27 | L45 A15 L49 A16 L52 L53 L54 A23 A26 of sketch 2 text T0 T2 T1 bodies 2 in component "Top"
component "Bottom" placed x (1, 0, 0) y (0, 1, 0) z (0, 0, 1) at (0, 0, 0)
component "Top" placed x (1, 0, 0) y (0, 1, 0) z (0, 0, 1) at (0, 0, 0)
